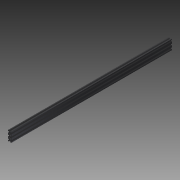
# Autodesk Inventor part: 20x60x1000mm
Saved by Autodesk Inventor 2014 SP1 (Build 180222100, 222)
## iProperties
Created: 2016-04-09
Part Number: 20x60x1000mm
Material: Generic
Document SubType Name: Modeling
Designer: Ben
Density: 1 g/cm^3
Appearance: Default
Author: Ben
Autodesk Inventor part; units mm, degrees
ref_plane "YZ Plane" through (0, 0, 0) normal (1, 0, 0) x (0, 1, 0)
ref_plane "XZ Plane" through (0, 0, 0) normal (0, 1, 0) x (-1, 0, 0)
ref_plane "XY Plane" through (0, 0, 0) normal (0, 0, 1) x (1, 0, 0)
sketch "Sketch1" plane through (0, 0, 0) normal (0, 0, 1) x (1, 0, 0)
  line L0 (-3.9007, 3.9007) -> (3.9007, 3.9007)
  line L1 (3.9007, 3.9007) -> (3.9007, -3.9007)
  line L2 (3.9007, -3.9007) -> (-3.9007, -3.9007)
  line L3 (-3.9007, -3.9007) -> (-3.9007, 3.9007)
  line L4 (0, 3.9007) -> (0, -3.9007) construction
  line L5 (-3.9007, 0) -> (3.9007, 0) construction
  circle A0 centre (0, 0) radius 2.1
  line L6 (0, 0) -> (-16.1173, 16.1173) construction
  line L7 (0, 0) -> (22.7933, 0) construction
  line L8 (-2.84, 3.9007) -> (-5.4993, 6.56)
  line L9 (-5.4993, 6.56) -> (-5.4993, 8.2)
  line L10 (-5.4993, 8.2) -> (-2.84, 8.2)
  line L11 (-2.84, 8.2) -> (-4.64, 10)
  line L12 (-4.64, 10) -> (-10, 10)
  line L13 (-10, 10) -> (-10, 4.64)
  line L14 (-10, 4.64) -> (-8.2, 2.84)
  line L15 (-8.2, 2.84) -> (-8.2, 5.4993)
  line L16 (-8.2, 5.4993) -> (-6.56, 5.4993)
  line L17 (-6.56, 5.4993) -> (-3.9007, 2.84)
  line L18 (-3.9007, 2.84) -> (-11.3102, 2.84) construction
  line L19 (-2.84, 3.9007) -> (-3.9007, 3.9007)
  line L20 (-3.9007, 2.84) -> (-3.9007, 3.9007)
  line L21 (-3.9007, -2.84) -> (-6.56, -5.4993)
  line L22 (-6.56, -5.4993) -> (-8.2, -5.4993)
  line L23 (-8.2, -5.4993) -> (-8.2, -2.84)
  line L24 (-8.2, -2.84) -> (-10, -4.64)
  line L25 (-10, -4.64) -> (-10, -10)
  line L26 (-10, -10) -> (-4.64, -10)
  line L27 (-4.64, -10) -> (-2.84, -8.2)
  line L28 (-2.84, -8.2) -> (-5.4993, -8.2)
  line L29 (-5.4993, -8.2) -> (-5.4993, -6.56)
  line L30 (-5.4993, -6.56) -> (-2.84, -3.9007)
  line L31 (-3.9007, -2.84) -> (-3.9007, -3.9007)
  line L32 (-2.84, -3.9007) -> (-3.9007, -3.9007)
  line L33 (2.84, -3.9007) -> (5.4993, -6.56)
  line L34 (5.4993, -6.56) -> (5.4993, -8.2)
  line L35 (5.4993, -8.2) -> (2.84, -8.2)
  line L36 (2.84, -8.2) -> (4.64, -10)
  line L37 (4.64, -10) -> (10, -10)
  line L38 (10, -10) -> (10, -4.64)
  line L39 (10, -4.64) -> (8.2, -2.84)
  line L40 (8.2, -2.84) -> (8.2, -5.4993)
  line L41 (8.2, -5.4993) -> (6.56, -5.4993)
  line L42 (6.56, -5.4993) -> (3.9007, -2.84)
  line L43 (2.84, -3.9007) -> (3.9007, -3.9007)
  line L44 (3.9007, -2.84) -> (3.9007, -3.9007)
  line L45 (3.9007, 2.84) -> (6.56, 5.4993)
  line L46 (6.56, 5.4993) -> (8.2, 5.4993)
  line L47 (8.2, 5.4993) -> (8.2, 2.84)
  line L48 (8.2, 2.84) -> (10, 4.64)
  line L49 (10, 4.64) -> (10, 10)
  line L50 (10, 10) -> (4.64, 10)
  line L51 (4.64, 10) -> (2.84, 8.2)
  line L52 (2.84, 8.2) -> (5.4993, 8.2)
  line L53 (5.4993, 8.2) -> (5.4993, 6.56)
  line L54 (5.4993, 6.56) -> (2.84, 3.9007)
  line L55 (3.9007, 2.84) -> (3.9007, 3.9007)
  line L56 (2.84, 3.9007) -> (3.9007, 3.9007)
  dimension "d7" = 4.2
  dimension "d8" = 135
  dimension "d9" = 1.5
  dimension "d10" = 1.64
  dimension "d11" = 1.8
  dimension "d12" = 2.84
  dimension "d13" = 10
  dimension "d16" = 360
  constraints: 114 end point, 10 parallel, 6 midpoint, 6 perpendicular, 4 equal length, 4 point on line, 2 horizontal, 1 centre point, 1 coincident, 99 other
  measures "d7" diameter of A0
  measures "d8" angle of L7 L6
  measures "d9" distance between parallel lines of L17 L8
  measures "d10" distance of L15.end L16.end
  measures "d11" distance between parallel lines of L13 L15
  measures "d12" distance from line of L5 L14.end
  measures "d13" distance between parallel lines of L5 L12
extrude "Extrusion1" add sketch "Sketch1" along normal blind 1000
pattern_linear "Rectangular Pattern1" count 3 spacing 20 along (0, -1, 0) of "Extrusion1"
sketch "Sketch2" plane through (0, 0, 1000) normal (0, 0, 1) x (1, 0, 0)
  line L0 (8.2, -2.84) -> (8.2, -5.4993) projected
  line L1 (8.2, -5.4993) -> (6.56, -5.4993) projected
  line L2 (-6.56, -5.4993) -> (-8.2, -5.4993) projected
  line L3 (-8.2, -5.4993) -> (-8.2, -2.84) projected
  line L4 (-8.2, -14.5007) -> (-6.56, -14.5007) projected
  line L5 (6.56, -14.5007) -> (8.2, -14.5007) projected
  line L6 (5.4993, -11.8) -> (5.4993, -13.44) projected
  line L7 (5.4993, -13.44) -> (2.84, -16.0993) projected
  line L8 (-2.84, -16.0993) -> (-5.4993, -13.44) projected
  line L9 (-5.4993, -8.2) -> (-5.4993, -6.56) projected
  line L10 (-5.4993, -6.56) -> (-2.84, -3.9007) projected
  line L11 (2.84, -3.9007) -> (5.4993, -6.56) projected
  line L12 (2.84, -8.2) -> (4.64, -10) projected
  line L13 (-8.2, -6.9993) -> (-5.9387, -6.9993)
  line L14 (-5.9387, -6.9993) -> (-4.1231, -5.1837)
  line L15 (-4.1231, -5.1837) -> (4.1231, -5.1837)
  line L16 (4.1231, -5.1837) -> (5.9387, -6.9993)
  line L17 (5.9387, -6.9993) -> (8.2, -6.9993)
  line L18 (8.2, -6.9993) -> (8.2, -13.0007)
  line L19 (8.2, -13.0007) -> (5.9387, -13.0007)
  line L20 (5.9387, -13.0007) -> (4.2461, -14.6932)
  line L21 (4.2461, -14.6932) -> (-4.2461, -14.6932)
  line L22 (-4.2461, -14.6932) -> (-5.9387, -13.0007)
  line L23 (-5.9387, -13.0007) -> (-8.2, -13.0007)
  line L24 (-8.2, -13.0007) -> (-8.2, -6.9993)
  dimension "d23" = 1.5
  dimension "d24" = 1.5
  dimension "d25" = 1.5
  dimension "d26" = 1.5
  constraints: 24 end point, 8 collinear, 8 perpendicular, 2 parallel
  measures "d23" distance between parallel lines of L2 L13
  measures "d24" distance between parallel lines of L1 L17
  measures "d25" distance between parallel lines of L5 L19
  measures "d26" distance between parallel lines of L4 L23
extrude "Extrusion2" cut sketch "Sketch2" against normal up to next
pattern_linear "Rectangular Pattern2" count 2 spacing 20 along (0, -1, 0) of "Extrusion2"
equation "\"d24\" = d23"
equation "\"d25\" = d23"
equation "\"d26\" = d23"
body "Solid1"
